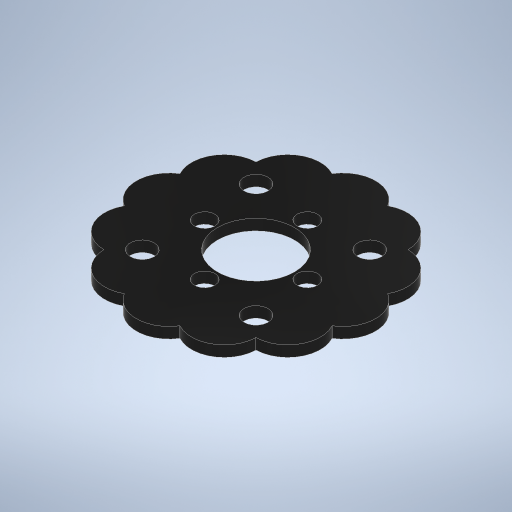
# Autodesk Inventor part: Motor Cap
Saved by Autodesk Inventor 2023.2 (Build 272271000, 271)
## iProperties
Created: 2022-12-29
Part Number: Motor Cap
Material: Nylon 6/6
Document SubType Name: Modeling
Designer: Nathan Cai
Density: 1.13 g/cm^3
Appearance: Smooth - Black
Mass: 1.4468 g
Surface Area: 19.2944 cm^2
Volume: 1.28035 cm^3
Author: Nathan Cai
Autodesk Inventor part; units mm, degrees
ref_plane "YZ Plane" through (0, 0, 0) normal (1, 0, 0) x (0, 1, 0)
ref_plane "XZ Plane" through (0, 0, 0) normal (0, 1, 0) x (-1, 0, 0)
ref_plane "XY Plane" through (0, 0, 0) normal (0, 0, 1) x (1, 0, 0)
sketch "Sketch1" plane through (0, 0, 0) normal (0, 1, 0) x (-1, 0, 0)
  circle A0 centre (0, 0) radius 5.625
  circle A1 centre (0, 0) radius 7.5 construction
  circle A2 centre (0, 0) radius 22.225 construction
  circle A3 centre (7.5, 0) radius 1.5
  line L0 (22.225, 0) -> (0, 0) construction
  circle A4 centre (0, 7.5) radius 1.5
  circle A5 centre (-7.5, 0) radius 1.5
  circle A6 centre (0, 0) radius 19.05
  circle A7 centre (0, -7.5) radius 1.5
  point P0 (0, 6)
  point P1 (6, 0)
  point P2 (0, -6)
  point P3 (-6, 0)
  dimension "d1" = 15
  dimension "d2" = 44.45
  dimension "d0" = 11.25
  dimension "d3" = 3
  dimension "d6" = 360
  dimension "d8" = 38.1
  constraints: 6 centre point, 4 coincident, 2 end point, 2 horizontal alignment, 1 horizontal, 1 point on line, 13 other
  measures "d0" diameter of A0
  measures "d3" diameter of A3
  measures "d8" diameter of A6
extrude "Extrusion1" add sketch "Sketch1" along normal blind 1.5875
sketch "Sketch2" plane through (0, 1.5875, 0) normal (0, 1, 0) x (1, 0, 0)
  circle A0 centre (0, 0) radius 11.75 construction
  line L0 (0, 0) -> (19.05, 0) construction
  circle A1 centre (0, 0) radius 19.05 projected
  line L1 (11.75, 0) -> (0, 0) construction
  line L2 (0, 0) -> (8.3085, -8.3085) construction
  circle A2 centre (8.3085, -8.3085) radius 1.7526
  circle A3 centre (8.3085, 8.3085) radius 1.7526
  circle A4 centre (-8.3085, 8.3085) radius 1.7526
  circle A5 centre (-8.3085, -8.3085) radius 1.7526
  dimension "d11" = 23.5
  dimension "d28" = 45
  dimension "d29" = 3.5052
  dimension "d32" = 360
  constraints: 6 end point, 5 centre point, 2 coincident, 2 horizontal, 2 point on circle, 1 horizontal alignment, 1 point on line, 10 other
  measures "d11" diameter of A0
  measures "d28" angle of L0 L2
  measures "d29" diameter of A2
extrude "Extrusion2" cut sketch "Sketch2" against normal through all contours A2 | A3 | A4 | A5
sketch "Sketch3" plane through (0, 1.5875, 0) normal (0, 1, 0) x (1, 0, 0)
  line L0 (0, 0) -> (12.7, 0) construction
  circle A0 centre (0, 0) radius 12.7 construction
  circle A1 centre (12.7, 0) radius 4.7625
  circle A2 centre (10.9985, 6.35) radius 4.7625
  circle A3 centre (6.35, 10.9985) radius 4.7625
  circle A4 centre (0, 12.7) radius 4.7625
  circle A5 centre (-6.35, 10.9985) radius 4.7625
  circle A6 centre (-10.9985, 6.35) radius 4.7625
  circle A7 centre (-12.7, 0) radius 4.7625
  circle A8 centre (-10.9985, -6.35) radius 4.7625
  circle A9 centre (-6.35, -10.9985) radius 4.7625
  circle A10 centre (0, -12.7) radius 4.7625
  circle A11 centre (6.35, -10.9985) radius 4.7625
  circle A12 centre (10.9985, -6.35) radius 4.7625
  circle A13 centre (0, 0) radius 19.05
  point P0 (11.1112, -11.1112)
  point P1 (4.067, -15.1781)
  point P2 (-4.067, -15.1781)
  point P3 (-11.1112, -11.1112)
  point P4 (-15.1781, -4.067)
  point P5 (-15.1781, 4.067)
  point P6 (-11.1112, 11.1112)
  point P7 (-4.067, 15.1781)
  point P8 (4.067, 15.1781)
  point P9 (11.1112, 11.1112)
  point P10 (15.1781, 4.067)
  point P11 (15.1781, -4.067)
  dimension "d19" = 25.4
  dimension "d20" = 9.525
  dimension "d23" = 360
  dimension "d25" = 38.1
  constraints: 13 centre point, 3 coincident, 2 end point, 1 horizontal, 1 horizontal alignment, 27 other
  measures "d20" diameter of A1
  measures "d25" diameter of A13
extrude "Extrusion3" cut sketch "Sketch3" against normal blind 25.4
body "Solid1"
